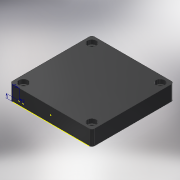
# Autodesk Inventor part: Ventillateur_60x60x11
Saved by Autodesk Inventor 2017 (Build 210142000, 142)
## iProperties
Part Number: Ventillateur_60x60x11
Material: Plastique ABS
Document SubType Name: Modeling
Designer: Adrien MARY
Density: 1.06 g/cm^3
Appearance: Lisse - Blanc(2)
Mass: 40.9927 g
Surface Area: 103.633 cm^2
Volume: 38.6724 cm^3
Stock Number: 1410-03-05
Project: 1410 LaserShow
Author: Adrien MARY
Autodesk Inventor part; units mm, degrees
ref_plane "YZ Plane" through (0, 0, 0) normal (1, 0, 0) x (0, 1, 0)
ref_plane "XZ Plane" through (0, 0, 0) normal (0, 1, 0) x (-1, 0, 0)
ref_plane "XY Plane" through (0, 0, 0) normal (0, 0, 1) x (1, 0, 0)
sketch "Esquisse1" plane through (0, 0, 0) normal (0, 0, 1) x (1, 0, 0)
  line L0 (-30, -30) -> (30, -30)
  line L1 (30, -30) -> (30, 30)
  line L2 (30, 30) -> (-30, 30)
  line L3 (-30, 30) -> (-30, -30)
  line L4 (-30, -30) -> (30, 30) construction
  line L5 (30, -30) -> (-30, 30) construction
  point P0 (0, 0)
  dimension "d0" = 60
  dimension "d1" = 60
  constraints: 12 end point, 2 midpoint, 2 parallel, 1 horizontal, 1 perpendicular
  measures "d0" distance of L2.end L1.end
  measures "d1" distance of L1.end L0.end
extrude "Extrusion1" add sketch "Esquisse1" along normal mid plane 11
sketch "Esquisse2" plane through (0, 0, 5.5) normal (0, 0, 1) x (1, 0, 0)
  point P0 (0, 0)
  point P1 (-25, 25)
  point P2 (25, 25)
  point P3 (25, -25)
  point P4 (-25, -25)
  dimension "d4" = 50
  dimension "d5" = 50
  dimension "d7" = 25
  dimension "d8" = 25
  constraints: 2 horizontal alignment, 2 vertical alignment
  measures "d4" distance of point (25, -25) point (-25, -25)
  measures "d5" distance of point (25, -25) point (25, 25)
  measures "d7" horizontal distance of point (25, 25) point (0, 0)
  measures "d8" horizontal distance of point (25, 25) point (0, 0)
hole "Perçage1" at (-25, 25, 5.5) at (25, 25, 5.5) at (25, -25, 5.5) at (-25, -25, 5.5) direction (0, 0, -1) diameter 4.4 end through all counterbore diameter 6.45 counterbore depth 3.16
fillet "Congé1" radius 2 4 edges at (-30, 30, 0) (30, 30, 0) (30, -30, 0) (-30, -30, 0)
sketch "Esquisse3" plane through (-28, -30, -5.5) normal (0, -1, 0) x (1, 0, 0)
  line L0 (56, 0) -> (0, 0) projected
  point P0 (28, 5.5)
  point P1 (5, 3)
  point P2 (8, 3)
  dimension "d17" = 3
  dimension "d18" = 3
  dimension "d19" = 5
  constraints: 1 horizontal alignment
  measures "d17" distance of point (5, 3) point (8, 3)
  measures "d18" distance from line of L0 point (5, 3)
  measures "d19" horizontal distance of L0.end point (5, 3)
equation "\"d7\" = 0.5 * d5"
equation "\"d8\" = 0.5 * d5"
equation "\"pi\" = 3.141593"
equation "\"nombredor\" = 1.61803"
